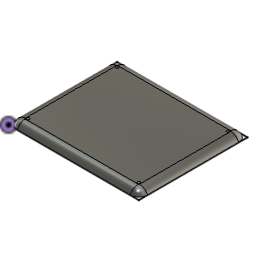
Open-Fluorometer-Lid v2 (Autodesk Fusion 360 design; units mm, degrees)
Autodesk Fusion 360 part; units mm, degrees
sketch "Sketch1" plane through (0, 0, 0) normal (0, 0, 1) x (1, 0, 0)
  line L0 (0, 0) -> (120, 0)
  line L1 (120, 0) -> (120, 100)
  line L2 (120, 100) -> (0, 100)
  line L3 (0, 100) -> (0, 0)
  dimension "d1" = 120
  dimension "d2" = 100
  constraint horizontal L0
  constraint vertical L1
  constraint horizontal L2
  constraint vertical L3
  constraint coincident L0.start L3.end
  measures "d1" distance of L0.start L0.end
  measures "d2" distance of L0.start L2.end
extrude "Extrude1" add sketch "Sketch1" along normal blind 5
fillet "Fillet1" radius 8 4 edges at (0, 0, 2.5) (0, 100, 2.5) (120, 0, 2.5) (120, 100, 2.5)
fillet "Fillet2" radius 8 8 edges at (117.6569, 97.6569, 5) (60, 100, 5) (2.3431, 97.6569, 5) (0, 50, 5) (2.3431, 2.3431, 5) (60, 0, 5) (117.6569, 2.3431, 5) (120, 50, 5)
sketch "Sketch2" plane through (0, 0, 5) normal (0, 0, 1) x (-1, 0, 0)
  line L0 (-112, -92.5838) -> (-8, -92.5838)
  arc A0 (-8, -92.5838) -> (-7.4162, -92) centre (-8, -92) ccw
  line L1 (-7.4162, -92) -> (-7.4162, -8)
  arc A1 (-7.4162, -8) -> (-8, -7.4162) centre (-8, -8) ccw
  line L2 (-8, -7.4162) -> (-112, -7.4162)
  arc A2 (-112, -7.4162) -> (-112.5838, -8) centre (-112, -8) ccw
  line L3 (-112.5838, -8) -> (-112.5838, -92)
  arc A3 (-112.5838, -92) -> (-112, -92.5838) centre (-112, -92) ccw
  line L4 (0, 0) -> (-9, 0)
  line L5 (-9, 0) -> (-9, -9)
  line L6 (-9, -9) -> (-111, -9)
  line L7 (-9, -9) -> (-9, -91)
  line L8 (-9, -91) -> (-111, -91)
  dimension "d9" = 9
  dimension "d10" = 9
  dimension "d11" = 102
  dimension "d12" = 82
  dimension "d14" = 102
  constraint coincident L4.start origin
  constraint parallel L2 L4
  constraint perpendicular L2 L5
  constraint perpendicular L3 L6
  constraint perpendicular L6 L7
  constraint perpendicular L7 L8
  measures "d9" distance of L4.start L4.end
  measures "d10" distance of L4.end L5.end
  measures "d11" distance of L5.end L6.end
  measures "d12" distance of L5.end L7.end
  measures "d14" distance of L7.end L8.end
hole "Hole1" at (111, 91, 5) direction (0, 0, -1) diameter 2.5 depth 5 tip angle 180
hole "Hole2" at (9, 91, 5) direction (0, 0, -1) diameter 2.5 depth 5 tip angle 180
hole "Hole3" at (9, 9, 5) direction (0, 0, -1) diameter 2.5 depth 5 tip angle 180
hole "Hole4" at (111, 9, 5) direction (0, 0, -1) diameter 2.5 depth 5 tip angle 180
